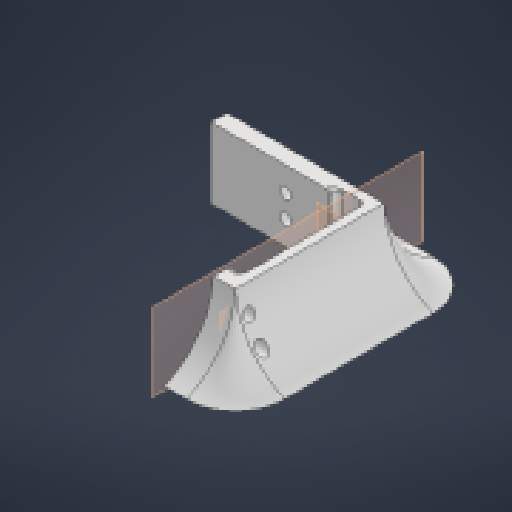
# Autodesk Inventor part: Base Side Armor - Left
Saved by Autodesk Inventor 2026.2 (Build 302298000, 298)
## iProperties
Created: 2024-09-28
Part Number: Base Side Armor - Left
Material: Generic
Document SubType Name: Modeling
Designer: Ethan
Density: 1 g/cm^3
Appearance: Default
Author: Ethan
Autodesk Inventor part; units mm, degrees
ref_plane "XZ Plane" through (0, 0, 0) normal (0, 1, 0) x (-1, 0, 0)
ref_plane "Back of Base Plane" through (0, 0, -70.0556) normal (0, 0, 1) x (1, 0, 0)
ref_plane "Side of Base Plane" through (6.5, 0, 0) normal (1, 0, 0) x (0, 1, 0)
ref_plane "Side Bolt Offset Plane" through (16.2, 0, 0) normal (1, 0, 0) x (0, 1, 0)
ref_plane "Back Bolt Offset Plane" through (0, 0, -78.0556) normal (0, 0, 1) x (1, 0, 0)
sketch "Interface - EDIT TO CHANGE SHAPE" plane through (0, 0, 0) normal (0, 1, 0) x (-1, 0, 0)
  line L0 (0, 0) -> (-14, 0) construction
  line L1 (-14, 0) -> (-14, -74.0556) construction
  line L2 (-14, -74.0556) -> (27.5, -74.0556) construction
  line L3 (27.5, -74.0556) -> (27.5, -70.0556) construction
  line L4 (-29.9, -70.0556) -> (46.4, -70.0556) construction
  line L5 (-14, -4.75) -> (-14, -74.0556)
  line L6 (-14, -74.0556) -> (2.7, -74.0556)
  line L7 (2.7, -74.0556) -> (2.7, -70.0556)
  line L8 (-19, 4.75) -> (-19, -79.0556)
  line L9 (-19, -79.0556) -> (35.5, -79.0556)
  line L10 (35.5, -79.0556) -> (35.5, -70.0556)
  line L11 (0, -95.8167) -> (0, 21.5111) construction
  line L12 (-14, -4.75) -> (-6.5, -4.75)
  line L13 (-19, 4.75) -> (-6.5, 4.75)
  line L14 (-6.5, 4.75) -> (-6.5, -4.75)
  line L15 (-6.5, -95.8167) -> (-6.5, 21.5111) construction
  line L16 (2.7, -70.0556) -> (35.5, -70.0556)
  dimension "d8" = 27.5
  dimension "d9" = 9.5
  dimension "d10" = 4
  dimension "d11" = 14
  dimension "d14" = 5
  dimension "d15" = 5
  dimension "d33" = 24.8
  dimension "d34" = 8
  constraints: 28 end point, 7 perpendicular, 4 collinear, 4 horizontal, 1 point on line, 1 vertical, 1 other
  measures "d8" distance between parallel lines of L11 L3
  measures "d9" distance of L13.end L12.end
  measures "d10" distance between parallel lines of L4 L2
  measures "d11" distance between parallel lines of L1 L11
  measures "d14" distance between parallel lines of L8 L5
  measures "d15" distance between parallel lines of L9 L6
  measures "d33" distance between parallel lines of L7 L3
  measures "d34" distance between parallel lines of L3 L10
extrude "Interface - EDIT TO CHANGE HEIGHT" add sketch "Interface - EDIT TO CHANGE SHAPE" along normal mid plane 40
sketch "Side Bolt Shaft Holes Sketch" plane through (16.2, 0, 0) normal (1, 0, 0) x (0, 1, 0)
  circle A0 centre (6.5, 0) radius 1.75
  circle A1 centre (-6.5, 0) radius 1.75
  line L0 (6.5, 0) -> (-6.5, 0) construction
  point P0 (0, 0)
  point P1 (0, 0)
  dimension "d18" = 6.5
  dimension "d19" = 3.5
  constraints: 3 coincident, 2 centre point, 2 end point, 1 equal radius, 1 horizontal, 1 midpoint
  measures "d18" distance of point (0, 0) A0.centre
  measures "d19" diameter of A0
extrude "Bolt Shaft Holes - Side" cut sketch "Side Bolt Shaft Holes Sketch" along normal blind 51.7 and the other way blind 12
sketch "Side Bolt Head Holes Sketch" plane through (16.2, 0, 0) normal (1, 0, 0) x (0, 1, 0)
  circle A0 centre (6.5, 0) radius 1.75 projected
  circle A1 centre (6.5, 0) radius 3.25
  circle A2 centre (-6.5, 0) radius 1.75 projected
  circle A3 centre (-6.5, 0) radius 3.25
  point P0 (0, 0)
  dimension "d22" = 6.5
  constraints: 2 centre point, 2 coincident, 1 equal radius
  measures "d22" diameter of A1
extrude "Bolt Head Holes - Side" cut sketch "Side Bolt Head Holes Sketch" along normal blind 6 contours A0 | A1 | A2 | A3
sketch "Back Bolt Shaft Holes Sketch" plane through (0, 0, -78.0556) normal (0, 0, 1) x (1, 0, 0)
  line L0 (-27.5, 6.5) -> (-27.5, -6.5) construction
  circle A0 centre (-27.5, 6.5) radius 1.75
  circle A1 centre (-27.5, -6.5) radius 1.75
  point P0 (0, 0)
  point P1 (-27.5, 0)
  point P2 (-27.5, 0)
  point P3 (-27.5, 0)
  point P4 (-27.5, 0)
  dimension "d25" = 6.5
  dimension "d26" = 3.5
  constraints: 3 coincident, 2 centre point, 2 end point, 1 equal radius, 1 midpoint, 1 vertical
  measures "d25" distance of point (-27.5, 0) L0.start
  measures "d26" diameter of A0
extrude "Bolt Shaft Holes - Back" cut sketch "Back Bolt Shaft Holes Sketch" against normal blind 30
sketch "Back Bolt Head Holes Sketch" plane through (0, 0, -78.0556) normal (0, 0, 1) x (1, 0, 0)
  circle A0 centre (-27.5, 6.5) radius 1.75 projected
  circle A1 centre (-27.5, 6.5) radius 3.25
  circle A2 centre (-27.5, -6.5) radius 3.25
  point P0 (0, 0)
  dimension "d29" = 6.5
  constraints: 2 centre point, 2 coincident, 1 equal radius
  measures "d29" diameter of A1
extrude "Bolt Head Holes - Back" cut sketch "Back Bolt Head Holes Sketch" against normal blind 40 contours A0 | A1 | A2
fillet "Mount Fillets" radius 2 4 edges at (10.25, 20, -4.75) (10.25, -20, -4.75) (-2.7, 20, -72.0556) (-2.7, -20, -72.0556)
fillet "Internal Fillets" radius 3 3 edges at (-2.7, 0, -74.0556) (14, 0, -74.0556) (14, 0, -4.75)
sketch "Sketch7" plane through (6.5, 20, 4.75) normal (0, 0, 1) x (1, 0, 0)
  line L0 (12.5, -40) -> (12.5, 0) projected
  arc A0 (12.5, 0) -> (40.2995, -40) centre (58.0152, 1.9723) ccw
  line L1 (12.5, -40) -> (40.2995, -40)
  point P0 (-6.5, -20)
  constraints: 2 end point, 2 point on circle, 1 centre point, 1 horizontal
sketch "Sketch8" plane through (19, -20, -79.0556) normal (1, 0, 0) x (0, 0, -1)
  line L0 (0, 0) -> (0, 40) projected
  line L1 (0, 0) -> (27.8, 0)
  arc A0 (0, 40) -> (27.8, 0) centre (45.5124, 41.9706) ccw
  point P0 (-79.0556, 20)
  dimension "d56" = 27.8
  dimension "d57" = 64.64
  constraints: 2 end point, 2 point on circle, 1 centre point, 1 horizontal
  measures "d56" distance of L0.start L1.end
sketch "Sketch9" plane through (19, -20, -79.0556) normal (1, 0, 0) x (0, 0, -1)
  line L0 (-83.8056, 0) -> (-83.8056, 40) projected
  arc A0 (-111.6056, 0) -> (-83.8056, 40) centre (-129.318, 41.9706) ccw
  line L1 (-111.6056, 0) -> (-83.8056, 0)
  point P0 (-79.0556, 20)
  dimension "d58" = 27.8
  dimension "d59" = 64.64
  constraints: 2 end point, 2 point on circle, 1 centre point, 1 horizontal
  measures "d58" distance of L1.start L0.start
extrude "Extrusion8" add sketch "Sketch8" against normal blind 54.5
extrude "Extrusion9" add sketch "Sketch7" against normal blind 83.806
extrude "Extrusion10" add sketch "Sketch9" against normal blind 12.5
sketch "Sketch10" plane through (19, 6.5, 0) normal (-1, 0, 0) x (0, 0, 1)
  circle A0 centre (0, 0) radius 3.25 projected
  circle A1 centre (0, -13) radius 3.25 projected
  point P0 (0, -6.5)
extrude "Extrusion11" cut sketch "Sketch10" against normal through all
sketch "Sketch11" plane through (-35.5, -20, -70.0556) normal (0, 0, 1) x (1, 0, 0)
  circle A0 centre (8, 26.5) radius 3.25 projected
  circle A1 centre (8, 13.5) radius 3.25 projected
  point P0 (35.5, 20)
extrude "Extrusion12" cut sketch "Sketch11" against normal through all
sketch "Sketch14" plane through (19, -20, 4.75) normal (0, 0, 1) x (1, 0, 0)
  line L0 (0, 40) -> (0, 0) projected
  line L1 (0, 0) -> (27.7995, 0) projected
  arc A0 (0, 40) -> (27.7995, 0) centre (45.5152, 41.9723) ccw projected
  point P0 (-19, 20)
revolve "Revolution1" add sketch "Sketch14" angle 90 about axis through (19, 20, 4.75) along (0, -1, 0)
sketch "Sketch15" plane through (19, -20, -79.056) normal (1, 0, 0) x (0, 0, -1)
  line L0 (0, 39.9908) -> (0, 0) projected
  line L1 (0, 0) -> (27.7996, 0) projected
  arc A0 (0, 39.9908) -> (27.7996, 0) centre (45.512, 41.9706) ccw projected
  point P0 (-79.056, 20)
revolve "Revolution2" add sketch "Sketch15" angle 90 about axis through (19, 19.9908, -79.056) along (0, -1, 0)
sketch "Sketch16" plane through (-35.5, -20, -70.0556) normal (-1, 0, 0) x (0, 0, 1)
  line L0 (0, 0) -> (0, 40) projected
  line L1 (0, 0) -> (-36.8, 0) projected
  arc A0 (-36.8, 0) -> (-9, 40) centre (-54.5124, 41.9706) ccw projected
  line L2 (-9, 40) -> (0, 40) projected
  point P0 (70.0556, 20)
extrude "Extrusion13" add sketch "Sketch16" along normal blind 34
body "Solid2"
